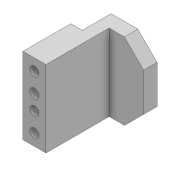
# Autodesk Inventor part: galvo_stop
Saved by Autodesk Inventor 2018.2 (Build 222227000, 227)
## iProperties
Created: 2018-07-18
Part Number: galvo_stop
Material: Generic
Document SubType Name: Modeling
Designer: legant_local
Density: 1 g/cm^3
Appearance: Default
Catalog Web Link: https://www.shapeways.com
Author: legant_local
Autodesk Inventor part; units mm, degrees
ref_plane "YZ Plane" through (0, 0, 0) normal (1, 0, 0) x (0, 1, 0)
ref_plane "XZ Plane" through (0, 0, 0) normal (0, 1, 0) x (-1, 0, 0)
ref_plane "XY Plane" through (0, 0, 0) normal (0, 0, 1) x (1, 0, 0)
sketch "Sketch1" plane through (0, 0, 0) normal (0, 0, 1) x (1, 0, 0)
  line L0 (-7.5, 10) -> (7.5, 10)
  line L1 (7.5, 10) -> (7.5, -10)
  line L2 (7.5, -10) -> (-7.5, -10)
  line L3 (-7.5, -10) -> (-7.5, 10)
  point P0 (0, 0)
  dimension "d0" = 15
  dimension "d1" = 20
  dimension "d2" = 7.5
  dimension "d3" = 10
  constraints: 8 end point, 2 parallel, 1 horizontal, 1 perpendicular
  measures "d0" distance of L1.end L2.end
  measures "d1" distance of L0.end L1.end
  measures "d2" distance from line of L1 point (0, 0)
  measures "d3" distance from line of L0 point (0, 0)
extrude "Extrusion1" add sketch "Sketch1" along normal blind 20
sketch "Sketch2" plane through (7.5, -10, 0) normal (1, 0, 0) x (0, 0, -1)
  line L0 (0, 20) -> (0, 0) projected
  line L1 (0, 20) -> (-20, 20) projected
  line L2 (-20, 0) -> (-20, 20) projected
  line L3 (0, 0) -> (-20, 0) projected
  line L4 (-20, 0) -> (0, 0)
  line L5 (0, 0) -> (0, 16.5)
  line L6 (0, 16.5) -> (-20, 16.5)
  line L7 (-20, 16.5) -> (-20, 0)
  point P0 (0, 10)
  dimension "d6" = 16.5
  constraints: 8 end point, 2 parallel, 1 horizontal, 1 perpendicular, 1 point on line
  measures "d6" distance between parallel lines of L3 L6
extrude "Extrusion2" cut sketch "Sketch2" against normal blind 9 contours L0 L3 L2 L6
sketch "Sketch3" plane through (-7.5, 10, 0) normal (0, 1, 0) x (1, 0, 0)
  circle A0 centre (3, -12) radius 0.7835
  circle A1 centre (3, -17) radius 0.7835
  line L0 (0, 0) -> (15, 0) projected
  line L1 (0, 0) -> (0, -20) projected
  line L2 (15, -20) -> (0, -20) projected
  line L3 (15, 0) -> (15, -20) projected
  circle A2 centre (3, -8) radius 0.7835
  circle A3 centre (3, -3) radius 0.7835
  point P0 (7.5, 0)
  dimension "d22" = 3
  dimension "d23" = 3
  dimension "d24" = 3
  dimension "d25" = 8
  dimension "d26" = 3
  dimension "d27" = 8
  dimension "d28" = 3
  dimension "d29" = 3
  constraints: 4 centre point
  measures "d22" distance from line of L1 A1.centre
  measures "d23" distance from line of L1 A0.centre
  measures "d24" distance from line of L2 A1.centre
  measures "d25" distance from line of L2 A0.centre
  measures "d26" distance from line of L0 A3.centre
  measures "d27" distance from line of L0 A2.centre
  measures "d28" distance from line of L1 A3.centre
  measures "d29" distance from line of L1 A2.centre
hole "Hole1" at (-4.5, 10, 12) at (-4.5, 10, 17) at (-4.5, 10, 8) at (-4.5, 10, 3) direction (0, -1, 0) diameter 2.4 end through all counterbore diameter 4.4 counterbore depth 7.5 clearance for "Socket Head Cap Screw" size "M2" standard "Ansi Metric M Profile"
sketch "Sketch4" plane through (-7.5, 10, 0) normal (0, 1, 0) x (1, 0, 0)
  arc A0 (2.0835, -10) -> (3.9165, -10) centre (3, -12) ccw projected
  circle A1 centre (3, -17) radius 2.2 projected
  line L0 (0, 0) -> (15, 0) projected
  line L1 (0, 0) -> (0, -20) projected
  line L2 (15, -20) -> (0, -20) projected
  line L3 (15, 0) -> (15, -20) projected
  line L4 (15, 0) -> (10, 0)
  line L5 (10, 0) -> (15, -5)
  line L6 (15, 0) -> (15, -5)
  line L7 (15, -20) -> (15, -15)
  line L8 (15, -20) -> (10, -20)
  line L9 (10, -20) -> (15, -15)
  arc A2 (3.9165, -10) -> (2.0835, -10) centre (3, -8) ccw projected
  point P0 (7.5, 0)
  dimension "d16" = 5
  dimension "d17" = 5
  dimension "d18" = 5
  dimension "d19" = 5
  constraints: 12 end point, 4 point on line
  measures "d16" distance of L0.end L4.end
  measures "d17" distance of L0.end L5.end
  measures "d18" distance of L2.start L7.end
  measures "d19" distance of L2.start L8.end
extrude "Extrusion3" cut sketch "Sketch4" against normal through all contours L0 L3 L5 | L9 L3 L2
sketch "Sketch5" plane through (-7.5, 10, 20) normal (0, 1, 0) x (1, 0, 0)
  line L0 (15, 15) -> (10, 20) projected
  line L1 (0, 20) -> (10, 20) projected
  line L2 (0, 20) -> (0, 0) projected
  line L3 (10, 0) -> (0, 0) projected
  line L4 (10, 0) -> (15, 5) projected
  line L5 (15, 15) -> (15, 5) projected
  circle A0 centre (3, 17) radius 2.2 projected
  circle A1 centre (3, 3) radius 2.2 projected
  arc A2 (3.9165, 10) -> (2.0835, 10) centre (3, 12) ccw projected
  arc A3 (2.0835, 10) -> (3.9165, 10) centre (3, 8) ccw projected
  line L6 (0, 20) -> (3, 20)
  line L7 (3, 20) -> (3, 0)
  line L8 (3, 0) -> (0, 0)
  line L9 (0, 0) -> (0, 20)
  point P0 (7.5, 20)
  dimension "d30" = 3
  constraints: 8 end point, 2 parallel, 1 horizontal, 1 perpendicular, 1 point on line
  measures "d30" distance of L7.end L8.end
extrude "Extrusion4" cut sketch "Sketch5" against normal blind 7.5 contours L7 A0 A2 A3 A1 L3 L2 L1 | L7 A0 | A1 L7 | L7 A3 A2 picked at (2.1729, 17.6329) picked at (2.3382, 2.4724) picked at (2.6945, 10)
equation "\"d2\" = 0.5 * d0"
equation "\"d3\" = 0.5 * d1"
body "Solid1"
